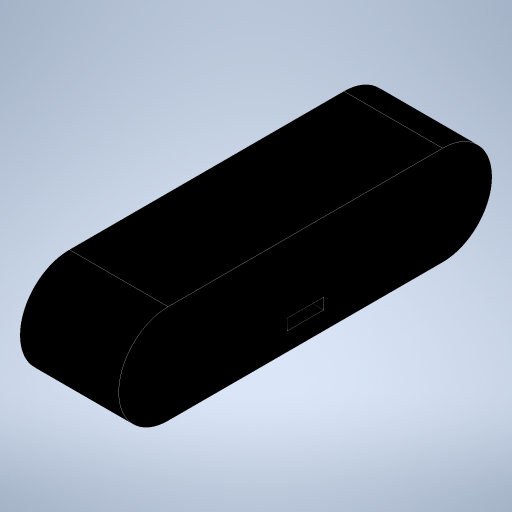
# Autodesk Inventor part: camera
Saved by Autodesk Inventor 2024 (Build 280153000, 153)
## iProperties
Created: 2024-05-02
Part Number: camera
Material: ABS プラスチック
Document SubType Name: Modeling
Designer: hirek
Density: 1.06 g/cm^3
Appearance: 黒
Mass: 85 g
Surface Area: 117.317 cm^2
Volume: 69.7581 cm^3
Author: hirek
Autodesk Inventor part; units mm, degrees
ref_plane "YZ Plane" through (0, 0, 0) normal (1, 0, 0) x (0, 1, 0)
ref_plane "XZ Plane" through (0, 0, 0) normal (0, 1, 0) x (-1, 0, 0)
ref_plane "XY Plane" through (0, 0, 0) normal (0, 0, 1) x (1, 0, 0)
sketch "スケッチ1" plane through (0, 0, 0) normal (0, 1, 0) x (-1, 0, 0)
  line L0 (0, 0) -> (27, 0)
  line L1 (27, 0) -> (27, -102)
  line L2 (27, -102) -> (0, -102)
  line L3 (0, -102) -> (0, 0)
  dimension "d0" = 27
  dimension "d1" = 102
  constraints: 8 end point, 2 parallel, 1 horizontal, 1 perpendicular
  measures "d0" distance of L1.end L2.end
  measures "d1" distance of L0.end L1.end
extrude "押し出し1" add sketch "スケッチ1" along normal blind 27
fillet "フィレット1" radius 13.5 4 edges at (-13.5, 27, 0) (-13.5, 0, 0) (-13.5, 27, -102) (-13.5, 0, -102)
sketch "スケッチ2" plane through (-27, 0, -88.5) normal (-1, 0, 0) x (0, 0, 1)
  line L0 (0, 27) -> (75, 27) projected
  line L1 (37.5, 27) -> (37.5, 0)
  line L2 (0, 0) -> (75, 0) projected
  circle A0 centre (37.5, 13.5) radius 6.5
  point P0 (88.5, 0)
  dimension "d5" = 13
  constraints: 3 midpoint, 2 end point, 1 centre point
  measures "d5" diameter of A0
extrude "押し出し2" cut sketch "スケッチ2" against normal blind 1
sketch "スケッチ3" plane through (0, 0, 0) normal (0, -1, 0) x (1, 0, 0)
  line L0 (-27, -88.5) -> (-27, -13.5) projected
  line L1 (-27, -51) -> (0, -51)
  line L2 (0, -13.5) -> (0, -88.5) projected
  point P0 (0, 0)
  point P1 (-13.5, -51)
  constraints: 3 midpoint, 2 end point
hole "穴1" at (-13.5, 0, -51) direction (0, 1, 0) diameter 6 depth 8 tip angle 118
sketch "スケッチ4" plane through (0, 0, -13.5) normal (1, 0, 0) x (0, 0, -1)
  line L0 (32.5, 8) -> (42.5, 8)
  line L1 (42.5, 8) -> (42.5, 5)
  line L2 (42.5, 5) -> (32.5, 5)
  line L3 (32.5, 5) -> (32.5, 8)
  line L4 (0, 0) -> (75, 0) projected
  point P0 (-13.5, 0)
  point P1 (37.5, 0)
  point P2 (37.5, 5)
  dimension "d15" = 10
  dimension "d16" = 3
  dimension "d17" = 5
  dimension "d18" = 0
  constraints: 8 end point, 2 midpoint, 2 parallel, 1 horizontal, 1 perpendicular
  measures "d15" distance of L1.end L2.end
  measures "d16" distance of L0.end L1.end
  measures "d17" distance between parallel lines of L4 L2
  measures "d18" horizontal distance of point (37.5, 0) point (37.5, 5)
extrude "押し出し3" cut sketch "スケッチ4" against normal blind 5
